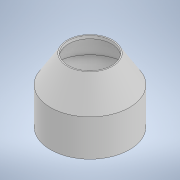
# Autodesk Inventor part: Top Nozzle Connector
Saved by Autodesk Inventor 2022 (Build 260153000, 153)
## iProperties
Created: 2023-01-19
Part Number: Top Nozzle Connector
Material: Generic
Document SubType Name: Modeling
Designer: ASUS
Density: 1 g/cm^3
Appearance: Default
Author: ASUS
Autodesk Inventor part; units mm, degrees
ref_plane "YZ Plane" through (0, 0, 0) normal (1, 0, 0) x (0, 1, 0)
ref_plane "XZ Plane" through (0, 0, 0) normal (0, 1, 0) x (-1, 0, 0)
ref_plane "XY Plane" through (0, 0, 0) normal (0, 0, 1) x (1, 0, 0)
sketch "Sketch1" plane through (0, 0, 0) normal (0, 1, 0) x (-1, 0, 0)
  circle A0 centre (0, 0) radius 16.2
  circle A1 centre (0, 0) radius 15
  dimension "d0" = 32.4
  dimension "d1" = 30
  constraints: 2 centre point, 2 coincident
  measures "d0" diameter of A0
  measures "d1" diameter of A1
extrude "Extrusion1" add sketch "Sketch1" along normal blind 15
sketch "Sketch2" plane through (0, 0, 0) normal (1, 0, 0) x (0, 1, 0)
  line L0 (25, 0) -> (25, -8.875) construction
  line L1 (15, -16.2) -> (15, 16.2) projected
  line L2 (15, -16.2) -> (15, -15)
  line L3 (25, -8.875) -> (15, -15)
  line L4 (26.2, -8.875) -> (26.2, -9.34)
  line L5 (15, -16.2) -> (26.2, -9.34)
  line L6 (25, -8.875) -> (26.2, -8.875)
  line L7 (15, 0) -> (31.8321, 0)
  point P0 (0, 0)
  dimension "d7" = 1.2
  constraints: 14 end point, 2 vertical, 1 horizontal, 1 midpoint, 1 perpendicular, 1 point on line
  measures "d7" distance of L1.start L2.end
revolve "Revolution1" add sketch "Sketch2" angle 360 about axis through (0, 15, 0) along (0, 1, 0)
body "Solid1"
